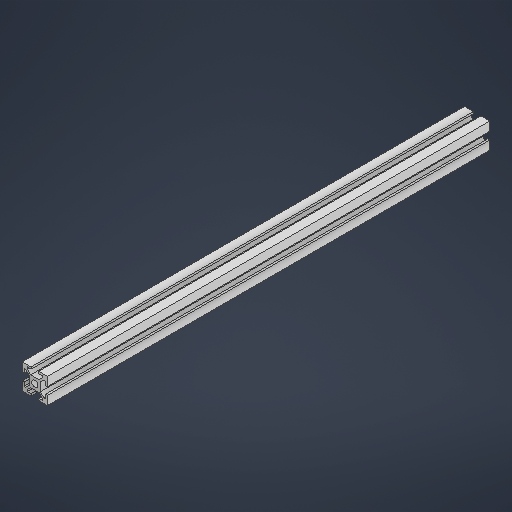
# Autodesk Inventor part: l350
Saved by Autodesk Inventor 2026.2 (Build 302298010, 298A)
## iProperties
Created: 2026-05-30
Part Number: l350
Material: 一般
Document SubType Name: Modeling
Designer: nyxeon
Density: 1 g/cm^3
Appearance: 既定
Author: nyxeon
Autodesk Inventor part; units mm, degrees
ref_plane "YZ Plane" through (0, 0, 0) normal (1, 0, 0) x (0, 1, 0)
ref_plane "XZ Plane" through (0, 0, 0) normal (0, 1, 0) x (-1, 0, 0)
ref_plane "XY Plane" through (0, 0, 0) normal (0, 0, 1) x (1, 0, 0)
sketch "スケッチ1" plane through (0, 0, 0) normal (0, 0, 1) x (1, 0, 0)
  circle A0 centre (0, 0) radius 2.5
  line L0 (-10, 10) -> (10, 10) construction
  line L1 (10, 10) -> (10, -10) construction
  line L2 (10, -10) -> (-10, -10) construction
  line L3 (-10, -10) -> (-10, 10) construction
  line L4 (-3, 10) -> (-3, 8.4) construction
  line L5 (-3, 8.4) -> (-6, 8.4) construction
  line L6 (-6, 8.4) -> (-6, 7.0607) construction
  line L7 (-6, 7.0607) -> (-3.3393, 4.4) construction
  line L8 (-3.3393, 4.4) -> (3.3393, 4.4) construction
  line L9 (3.3393, 4.4) -> (6, 7.0607) construction
  line L10 (6, 7.0607) -> (6, 8.4) construction
  line L11 (6, 8.4) -> (3, 8.4) construction
  line L12 (3, 8.4) -> (3, 10) construction
  line L13 (-10, 10) -> (10, -10) construction
  line L14 (-10, 10) -> (-3, 10)
  line L15 (-3, 10) -> (-3, 8.4)
  line L16 (-3, 8.4) -> (-6, 8.4)
  line L17 (-6, 8.4) -> (-6, 7.0607)
  line L18 (-6, 7.0607) -> (-3.3393, 4.4)
  line L19 (-3.3393, 4.4) -> (3.3393, 4.4)
  line L20 (3.3393, 4.4) -> (6, 7.0607)
  line L21 (6, 7.0607) -> (6, 8.4)
  line L22 (6, 8.4) -> (3, 8.4)
  line L23 (3, 8.4) -> (3, 10)
  line L24 (3, 10) -> (10, 10)
  line L25 (-10, -10) -> (-10, -3)
  line L26 (-10, -3) -> (-8.4, -3)
  line L27 (-8.4, -3) -> (-8.4, -6)
  line L28 (-8.4, -6) -> (-7.0607, -6)
  line L29 (-7.0607, -6) -> (-4.4, -3.3393)
  line L30 (-4.4, -3.3393) -> (-4.4, 3.3393)
  line L31 (-4.4, 3.3393) -> (-7.0607, 6)
  line L32 (-8.4, 6) -> (-8.4, 3)
  line L33 (-7.0607, 6) -> (-8.4, 6)
  line L34 (-8.4, 3) -> (-10, 3)
  line L35 (-10, 3) -> (-10, 10)
  line L36 (10, -10) -> (3, -10)
  line L37 (3, -10) -> (3, -8.4)
  line L38 (3, -8.4) -> (6, -8.4)
  line L39 (6, -8.4) -> (6, -7.0607)
  line L40 (6, -7.0607) -> (3.3393, -4.4)
  line L41 (3.3393, -4.4) -> (-3.3393, -4.4)
  line L42 (-3.3393, -4.4) -> (-6, -7.0607)
  line L43 (-6, -8.4) -> (-3, -8.4)
  line L44 (-6, -7.0607) -> (-6, -8.4)
  line L45 (-3, -8.4) -> (-3, -10)
  line L46 (-3, -10) -> (-10, -10)
  line L47 (10, 10) -> (10, 3)
  line L48 (10, 3) -> (8.4, 3)
  line L49 (8.4, 3) -> (8.4, 6)
  line L50 (8.4, 6) -> (7.0607, 6)
  line L51 (7.0607, 6) -> (4.4, 3.3393)
  line L52 (4.4, 3.3393) -> (4.4, -3.3393)
  line L53 (4.4, -3.3393) -> (7.0607, -6)
  line L54 (8.4, -6) -> (8.4, -3)
  line L55 (7.0607, -6) -> (8.4, -6)
  line L56 (8.4, -3) -> (10, -3)
  line L57 (10, -3) -> (10, -10)
  point P0 (-10, 0)
  point P1 (0, 10)
  dimension "d0" = 20
  dimension "d1" = 20
  dimension "d2" = 6
  dimension "d3" = 3
  dimension "d4" = 1.6
  dimension "d5" = 4
  dimension "d6" = 12
  dimension "d7" = 6
  dimension "d8" = 135
  dimension "d9" = 135
  dimension "d10" = 0.75
  dimension "d11" = 5
  dimension "d14" = 360
  constraints: 116 end point, 12 point on line, 9 perpendicular, 5 parallel, 2 horizontal, 2 midpoint, 1 centre point, 1 coincident, 1 horizontal alignment, 1 vertical alignment, 93 other
  measures "d0" distance of L0.start L0.end
  measures "d1" distance of L0.end L1.end
  measures "d2" distance between parallel lines of L12 L4
  measures "d3" distance from line of point (0, 10) L12
  measures "d4" distance of L11.end L12.end
  measures "d5" distance between parallel lines of L8 L11
  measures "d6" distance of L10.end L5.end
  measures "d7" distance from line of point (0, 10) L6
  measures "d8" angle of L8 L7
  measures "d9" angle of L9 L8
  measures "d10" distance between parallel lines of L13 L7
  measures "d11" diameter of A0
extrude "押し出し1" add sketch "スケッチ1" along normal mid plane 350
equation "\"d7\" = 0.5 * d6"
equation "\"d9\" = d8"
